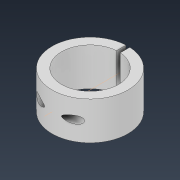
# Autodesk Inventor part: 0311_練習2
Saved by Autodesk Inventor 2022 (Build 260153000, 153)
## iProperties
Created: 2022-03-11
Part Number: 0311_練習2
Material: 一般
Document SubType Name: Modeling
Designer: user
Density: 1 g/cm^3
Appearance: 預設
Author: user
Autodesk Inventor part; units mm, degrees
ref_plane "YZ Plane" through (0, 0, 0) normal (1, 0, 0) x (0, 1, 0)
ref_plane "XZ Plane" through (0, 0, 0) normal (0, 1, 0) x (-1, 0, 0)
sketch "草圖1" plane through (0, 0, 0) normal (0, 1, 0) x (-1, 0, 0)
  circle A0 centre (0, 0) radius 15
  circle A1 centre (0, 0) radius 20
  dimension "d0" = 30
  dimension "d1" = 5
  constraints: 2 centre point, 1 coincident
  measures "d0" diameter of A0
  measures "d1" radial gap between concentric circles of A0 A1
extrude "擠出1" add sketch "草圖1" along normal mid plane 20
sketch "草圖2" plane through (0, 0, 0) normal (0, 0, 1) x (1, 0, 0)
  circle A0 centre (0, 0) radius 3
  dimension "d4" = 6
  constraints: 1 centre point, 1 coincident
  measures "d4" diameter of A0
sketch "草圖3" plane through (0, 0, 0) normal (0, 0, 1) x (1, 0, 0)
  line L0 (-20, -10) -> (20, -10) projected
  line L1 (20, 10) -> (-20, 10) projected
  circle A0 centre (17.5034, 0) radius 1
  line L2 (20, 10) -> (20, -10)
  line L3 (20, -10) -> (20, 10) projected
  line L4 (20, 10) -> (-20, 10) projected
  line L5 (15.0068, 10) -> (20, 10)
  point P0 (0, 0)
  point P1 (20, 0)
  point P2 (17.5034, 10)
  dimension "d5" = 2
  constraints: 4 end point, 2 collinear, 2 midpoint, 1 centre point, 1 horizontal alignment, 1 point on line, 1 vertical alignment
  measures "d5" diameter of A0
extrude "擠出2" cut sketch "草圖3" along normal through all both and the other way through all
sketch "草圖4" plane through (0, 0, 0) normal (0, 1, 0) x (-1, 0, 0)
  circle A0 centre (0, 0) radius 20 projected
  circle A1 centre (0, 0) radius 15 projected
  circle A2 centre (0, 0) radius 20 projected
  line L0 (19.975, -1) -> (14.9666, -1)
  circle A3 centre (0, 0) radius 15 projected
  line L1 (28, 0) -> (-28, 0) projected
  line L2 (19.975, 1) -> (14.9666, 1)
  dimension "d8" = 1
  constraints: 4 end point, 2 symmetric about line, 1 horizontal, 4 other
  measures "d8" distance between parallel lines of L1 L0
extrude "擠出3" cut sketch "草圖4" along normal through all both and the other way through all contours L1 A1 L2 A0 | A0 L0 A1 L1 picked at (16.6568, 0.5558) picked at (16.6568, -0.5558)
ref_plane "工作平面1" through (0, 0, 3) normal (0, 0, 1) x (1, 0, 0)
sketch "草圖5" plane through (0, 0, 3) normal (0, 0, 1) x (1, 0, 0)
  line L0 (-19.975, 10) -> (-19.975, -10) projected
  line L1 (-19.975, -10) -> (-19.975, -10) projected
  line L2 (-19.975, -10) -> (-19.975, 10) projected
  line L3 (-19.975, 10) -> (-19.975, 10) projected
  spline S0 degree 5 poles (16.5034, 0) (16.5037, -0.3304) (16.6391, -0.6617) (16.9151, -0.9151) (17.5618, -1.1213) (18.1683, -0.8385) (18.3912, -0.5976) (18.6137, -0.0031) (18.395, 0.593) (18.1721, 0.8363) (17.5647, 1.1217) (16.9159, 0.9158) (16.6393, 0.6625) (16.5037, 0.3307) (16.5034, 0) knots 0 0 0 0 0 0 0.26304 0.26304 0.26304 0.499355 0.499355 0.499355 0.736707 0.736707 0.736707 1 1 1 1 1 1 projected
  line L4 (19.7737, 10) -> (19.7737, -10) projected
  line L5 (19.7737, -10) -> (14.6969, -10) projected
  line L6 (14.6969, -10) -> (14.6969, 10) projected
  line L7 (14.6969, 10) -> (19.7737, 10) projected
  circle A0 centre (17.5034, 0) radius 1 projected
  line L8 (-19.7737, -10) -> (-19.7737, 10) projected
  line L9 (-19.7737, 10) -> (-14.6969, 10) projected
  line L10 (-14.6969, 10) -> (-14.6969, -10) projected
  line L11 (-14.6969, -10) -> (-19.7737, -10) projected
  line L12 (14.6969, 10) -> (19.7737, 10)
  line L13 (19.7737, 10) -> (19.7737, -10)
  line L14 (19.7737, -10) -> (14.6969, -10)
  line L15 (14.6969, -10) -> (14.6969, 10)
  circle A1 centre (17.5034, 0) radius 2
  point P0 (0, 0)
  point P1 (18.3303, -0.5624)
  point P2 (19.7737, 0)
  point P3 (17.2353, 10)
  dimension "d15" = 4
  constraints: 8 end point, 2 midpoint, 2 parallel, 1 centre point, 1 coincident, 1 horizontal, 1 perpendicular, 2 other
  measures "d15" diameter of A1
extrude "擠出5" cut sketch "草圖5" along normal through all both and the other way through all contours A1
